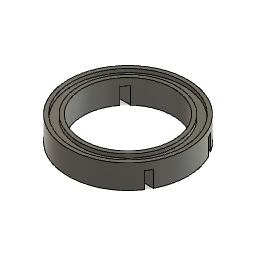
lager v2 (Autodesk Fusion 360 design; units mm, degrees)
Autodesk Fusion 360 part; units mm, degrees
sketch "Sketch1" plane through (0, 0, 0) normal (0, 1, 0) x (1, 0, 0)
  circle A0 centre (0, 0) radius 26.5
  circle A1 centre (0, 0) radius 32.5
  circle A2 centre (0, 0) radius 24.5
  circle A3 centre (0, 0) radius 30.5
  line L0 (-45.2216, 18) -> (54.7784, 18)
  line L1 (54.7784, 18) -> (54.7784, 15)
  line L2 (54.7784, 15) -> (-45.2216, 15)
  line L3 (-45.2216, 15) -> (-45.2216, 18)
  line L4 (-43, -15) -> (50, -15)
  line L5 (50, -15) -> (50, -18)
  line L6 (50, -18) -> (-43, -18)
  line L7 (-43, -18) -> (-43, -15)
  dimension "d1" = 53
  dimension "d2" = 65
  dimension "d3" = 49
  dimension "d4" = 61
  dimension "d10" = 100
  dimension "d11" = 3
  dimension "d12" = 15
  dimension "d13" = 93
  dimension "d14" = 3
  dimension "d15" = 15
  constraint coincident A0.centre A1.centre
  constraint concentric A0 A1
  constraint concentric A0 A3
  constraint horizontal L0
  constraint vertical L1
  constraint horizontal L2
  constraint vertical L3
  constraint horizontal L4
  constraint vertical L5
  constraint horizontal L6
  constraint vertical L7
  measures "d1" diameter of A0
  measures "d2" diameter of A1
  measures "d3" diameter of A2
  measures "d4" diameter of A3
  measures "d10" distance of L0.start L0.end
  measures "d11" distance of L0.start L2.end
  measures "d12" distance of A0.centre L2
  measures "d13" distance of L4.start L4.end
  measures "d14" distance of L4.start L6.end
  measures "d15" distance of A0.centre L4
extrude "Extrude3" add sketch "Sketch1" along normal blind 11 contours A0 A3 L2 L4 | A0 A3 L0 L2 | A0 A3 L4 L6 | A0 A3 L0 | A2 L0 L2 | A2 L2 L4 | A0 A3 L6 | A2 L4 L6 | A0 A3 L0 L2 | A2 L0 | A0 A3 L4 L6 | A2 L6 | A0 A3 L2 L4 makes body 1 at (6.1722, 11, 13.8445) makes body 2 at (30.3484, 3.6667, 3.0368)
extrude "Extrude4" add sketch "Sketch1" along normal blind 13 contours A0 A2 L2 L4 | A0 A2 L0 L2 | A0 A2 L4 L6 | A0 A2 L0 | A1 A3 L2 L4 | A1 A3 L0 L2 | A0 A2 L6 | A1 A3 L4 L6 | A0 A2 L0 L2 | A1 A3 L0 | A0 A2 L2 L4 | A0 A2 L4 L6 | A1 A3 L6 | A1 A3 L0 L2 | A1 A3 L4 L6 | A1 A3 L2 L4 bodies 1 2
extrude "Extrude5" cut sketch "Sketch1" along normal blind 9 contours A0 A2 L0 L2 | A0 A3 L0 L2 | A0 A3 L4 L6 | A0 A2 L4 L6 | A1 A3 L0 L2 | A2 L0 L2 | A2 L4 L6 | A1 A3 L4 L6 | A0 A2 L0 L2 | A0 A3 L0 L2 | A0 A3 L4 L6 | A0 A2 L4 L6 | A1 A3 L0 L2 | A1 A3 L4 L6 | A1 L0 L2 L3 | A1 L4 L6 L7 bodies 1
extrude "Extrude6" cut 1 faces at (6.1722, 11, 13.8445) along direction (0, -1, 0) blind 29 on bodies 1 bodies 1
equation "d3 = 24.5 * 2 mm"
